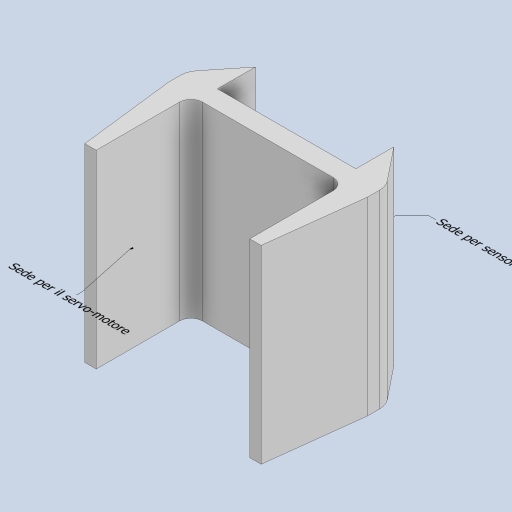
# Autodesk Inventor part: Sensore prossimale
Saved by Autodesk Inventor 2023.2 (Build 272271030, 271C)
## iProperties
Created: 2023-02-07
Part Number: Sensore prossimale
Material: Generico
Document SubType Name: Modeling
Designer: daler
Density: 1 g/cm^3
Appearance: Default
Author: daler
Autodesk Inventor part; units mm, degrees
ref_plane "YZ Plane" through (0, 0, 0) normal (1, 0, 0) x (0, 1, 0)
ref_plane "XZ Plane" through (0, 0, 0) normal (0, 1, 0) x (-1, 0, 0)
ref_plane "XY Plane" through (0, 0, 0) normal (0, 0, 1) x (1, 0, 0)
sketch "Schizzo1" plane through (0, 0, 0) normal (0, 0, 1) x (1, 0, 0)
  line L0 (-10.5, 10) -> (10.5, 10)
  line L1 (10.5, 10) -> (10.5, -10)
  line L2 (10.5, -10) -> (-10.5, -10)
  line L3 (-10.5, -10) -> (-10.5, 10)
  line L4 (-10.5, 10) -> (10.5, -10) construction
  line L5 (10.5, 10) -> (-10.5, -10) construction
  line L6 (-7.3, 10) -> (-7.3, -10)
  line L7 (7.3, 10) -> (7.3, -10)
  line L8 (8.1, -10) -> (8.1, 10)
  line L9 (-8.1, -10) -> (-8.1, 10)
  point P0 (0, 0)
  point P1 (0, 0)
  dimension "d0" = 21
  dimension "d1" = 20
  dimension "d2" = 3.2
  dimension "d3" = 3.2
  dimension "d17" = 2.4
  dimension "d19" = 2.4
  constraints: 20 end point, 8 point on line, 5 perpendicular, 2 parallel, 1 coincident, 1 horizontal, 1 midpoint
  measures "d0" distance of L0.start L0.end
  measures "d1" distance of L2.end L0.start
  measures "d2" distance between parallel lines of L3 L6
  measures "d3" distance between parallel lines of L1 L7
  measures "d17" distance between parallel lines of L3 L9
  measures "d19" distance between parallel lines of L1 L8
extrude "Estrusione4" add sketch "Schizzo1" along normal blind 2
extrude "Estrusione5" add sketch "Schizzo1" against normal blind 4 contours L0 L9 L2 L3 | L0 L6 L2 L9 | L0 L8 L2 L7 | L0 L1 L2 L8
extrude "Estrusione6" add sketch "Schizzo1" along normal blind 12 contours L0 L9 L2 L3 | L0 L1 L2 L8
fillet "Raccordo1" radius 1.2 2 edges at (8.1, 0, 2) (-8.1, 0, 2)
sketch "Schizzo3" plane through (-7.3, 10, 0) normal (0, 1, 0) x (1, 0, 0)
  line L0 (-3.2, 4) -> (-3.2, -12) projected
  line L1 (0, 4) -> (-3.2, 4) projected
  line L2 (-3.2, 0) -> (0, 4)
  line L3 (0, 4) -> (0, 0)
  line L4 (0, 0) -> (-3.2, 0)
  line L5 (14.6, 4) -> (17.8, 4) projected
  line L6 (14.6, 4) -> (17.8, 0)
  line L7 (17.8, 4) -> (17.8, -12) projected
  line L8 (14.6, 0) -> (14.6, 4)
  line L9 (14.6, 0) -> (17.8, 0)
  line L10 (-3.2, 0) -> (-3.2, 4)
  line L11 (0, 4) -> (-3.2, 4)
  line L12 (14.6, 4) -> (17.8, 4)
  line L13 (17.8, 0) -> (17.8, 4)
  point P0 (7.3, 0)
  constraints: 20 end point, 6 perpendicular, 5 point on line, 1 collinear, 1 vertical
extrude "Estrusione7" cut sketch "Schizzo3" against normal blind 100 contours L1 L2 L0 | L5 L7 L6
fillet "Raccordo2" radius 2 2 edges at (-10.5, 0, 0) (10.5, 0, 0)
sketch "Schizzo4" plane through (-7.3, 10, 0) normal (0, 1, 0) x (1, 0, 0)
  line L0 (-3.2, -0.7016) -> (-3.2, -12) projected
  line L1 (-3.2, -1.9701) -> (-2, -12)
  line L2 (-0.8, -12) -> (-3.2, -12) projected
  line L3 (-2, -12) -> (-3.2, -12)
  line L4 (-3.2, -1.9701) -> (-3.2, -12)
  point P0 (7.3, 0)
  constraints: 6 end point, 2 perpendicular, 1 midpoint, 1 point on line
extrude "Estrusione8" cut sketch "Schizzo4" against normal blind 100
mirror "Specchio1" about plane through (0, 0, 0) normal (1, 0, 0) of "Estrusione8"
